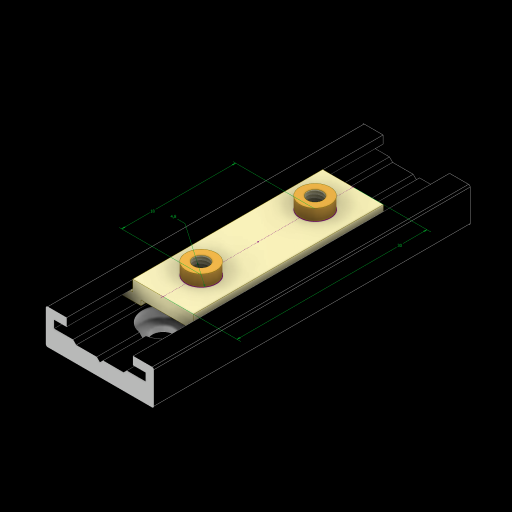
# Autodesk Inventor part: NS-17_IGUS-Fpührung
Saved by Autodesk Inventor 2024 (Build 280153000, 153)
## iProperties
Created: 2023-10-20
Part Number: NS-17_IGUS-Fpührung
Material: Aluminium 6061
Document SubType Name: Modeling
Designer: buchmannmartin
Mass: 7.82276 g
Surface Area: 30.3585 cm^2
Volume: 2.89732 cm^3
Density: 2.7 g/cm^3
Appearance: Eloxiert - Schwarz
Author: buchmannmartin
Autodesk Inventor part; units mm, degrees
ref_plane "YZ Plane" through (0, 0, 0) normal (1, 0, 0) x (0, 1, 0)
ref_plane "XZ Plane" through (0, 0, 0) normal (0, 1, 0) x (-1, 0, 0)
ref_plane "XY Plane" through (0, 0, 0) normal (0, 0, 1) x (1, 0, 0)
sketch "Skizze1" plane through (0, 0, 0) normal (0, 0, 1) x (1, 0, 0)
  line L0 (-8.5, -5.5) -> (8.5, -5.5)
  line L1 (8.5, -5.5) -> (8.5, 0)
  line L2 (8.5, 0) -> (5.25, 0)
  line L3 (5.25, 0) -> (5.25, -1.25)
  line L4 (5.25, -1.25) -> (7.25, -1.25)
  line L5 (7.25, -1.25) -> (7.25, -2.5)
  line L6 (7.25, -2.5) -> (4.25, -2.5)
  line L7 (4.25, -2.5) -> (3.75, -3)
  line L8 (3.75, -3) -> (0.5, -3)
  line L9 (0.5, -3) -> (0, -3.5)
  line L10 (0, 0) -> (0, -5.5) construction
  line L11 (-8.5, 0) -> (-5.25, 0)
  line L12 (-5.25, 0) -> (-5.25, -1.25)
  line L13 (-5.25, -1.25) -> (-7.25, -1.25)
  line L14 (-7.25, -1.25) -> (-7.25, -2.5)
  line L15 (-7.25, -2.5) -> (-4.25, -2.5)
  line L16 (-4.25, -2.5) -> (-3.75, -3)
  line L17 (-3.75, -3) -> (-0.5, -3)
  line L18 (-0.5, -3) -> (0, -3.5)
  line L19 (-8.5, 0) -> (-8.5, -5.5)
  line L20 (-5.25, -1.25) -> (-4.8, -1.25)
  line L21 (-4.8, -1.25) -> (-4.8, 0.5)
  line L22 (-4.8, 0.5) -> (4.8, 0.5)
  line L23 (4.8, 0.5) -> (4.8, -1.25)
  line L24 (4.8, -1.25) -> (5.25, -1.25)
  line L25 (-4.25, -2.5) -> (-3.5, -2.5)
  line L26 (-3.5, -2.5) -> (-3.5, -1.7)
  line L27 (-3.5, -1.7) -> (3.5, -1.7)
  line L28 (3.5, -1.7) -> (3.5, -2.5)
  line L29 (3.5, -2.5) -> (4.25, -2.5)
  point P0 (0, 0.5)
  point P1 (0, -1.7)
  dimension "d0" = 17
  dimension "d1" = 5.5
  dimension "d2" = 3
  dimension "d3" = 2.5
  dimension "d4" = 7.5
  dimension "d5" = 14.5
  dimension "d6" = 10.5
  dimension "d8" = 1.25
  dimension "d9" = 1.25
  dimension "d13" = 9.6
  dimension "d14" = 6
  dimension "d15" = 7
  dimension "d16" = 2.2
  constraints: 60 end point, 15 perpendicular, 8 symmetric about line, 6 point on line, 3 horizontal, 3 midpoint, 3 parallel, 2 vertical
  measures "d0" distance of L0.start L0.end
  measures "d1" distance between parallel lines of L0 L2
  measures "d2" distance between parallel lines of L0 L6
  measures "d3" distance between parallel lines of L0 L8
  measures "d4" distance of L7.end L16.end
  measures "d5" distance between parallel lines of L5 L14
  measures "d6" distance between parallel lines of L3 L12
  measures "d8" distance between parallel lines of L19 L14
  measures "d9" distance of L12.start L12.end
  measures "d13" distance between parallel lines of L23 L21
  measures "d14" distance between parallel lines of L0 L22
  measures "d15" distance of L26.end L27.end
  measures "d16" distance between parallel lines of L22 L27
extrude "Extrusion1" add sketch "Skizze1" along normal mid plane 50 contours L19 L11 L12 L13 L14 L15 L16 L17 L18 L9 L8 L7 L6 L5 L4 L3 L2 L1 L0
fillet "Rundung1" radius 0.25 4 edges at (-8.5, 0, 0) (8.5, 0, 0) (8.5, -5.5, 0) (-8.5, -5.5, 0)
extrude "Extrusion2" add sketch "Skizze1" along normal mid plane 30 separate body contours L20 L21 L22 L23 L24 L4 L5 L6 L29 L28 L27 L26 L25 L15 L14 L13
sketch "Skizze2" plane through (-4.8, 0.5, 15) normal (0, 1, 0) x (1, 0, 0)
  line L0 (4.8, 6) -> (4.8, 24) construction
  circle A0 centre (4.8, 6) radius 2.4
  circle A1 centre (4.8, 24) radius 2.4
  line L1 (4.8, 30) -> (4.8, 0) construction
  point P0 (4.8, 15)
  point P1 (4.8, 15)
  dimension "d19" = 18
  dimension "d20" = 4.8
  dimension "d30" = 30
  constraints: 4 end point, 3 coincident, 2 centre point, 2 midpoint, 2 vertical, 1 equal radius
  measures "d19" distance of L0.start L0.end
  measures "d20" diameter of A0
  measures "d30" distance of L1.start L1.end
extrude "Extrusion3" add sketch "Skizze2" along normal blind 1.8 bodies 2
hole "Bohrung1" at (0, 0.5, 9) at (0, 0.5, -9) direction (0, -1, 0) diameter 2.459 end through all start extended yes bodies 2 thread size "M3x0.5" class "6H" standard "ISO Metric profile"
hole "Bohrung2" at (0, 0.5, -15) at (0, 0.5, 15) direction (0, -1, 0) diameter 3.4 end through all counterbore diameter 6.5 counterbore depth 5.1 bodies 1 clearance for "Inbusschraube ISO 4762" size "M3" standard "ISO"
equation "\"d9\" = d8"
